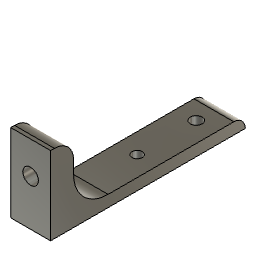
L Bracket v3 (Autodesk Fusion 360 design; units mm, degrees)
Autodesk Fusion 360 part; units mm, degrees
note: some values were not read from the file. Set by a fixed rule: which sketch regions a step uses.
sketch "Sketch1" plane through (0, 0, 0) normal (1, 0, 0) x (0, 1, 0)
  line L0 (0, 0) -> (0, 51)
  line L1 (0, 0) -> (127, 0)
  line L2 (127, 0) -> (127, 0.0001)
  line L3 (0, 51) -> (2.5, 51)
  line L4 (37.5, 7.5) -> (119.5, 7.5)
  line L5 (-5, 0) -> (-5, 33)
  line L6 (69.5, -10) -> (108, -10)
  line L7 (15, 30) -> (15, 38.5)
  arc A0 (15, 38.5) -> (2.5, 51) centre (2.5, 38.5) ccw
  arc A1 (127, 0.0001) -> (119.5, 7.5) centre (119.5, 0) ccw
  arc A2 (15, 30) -> (37.5, 7.5) centre (37.5, 30) ccw
  point P0 (126.9999, 7.5)
  point P1 (15, 51)
  point P2 (15, 7.5)
  dimension "d1" = 51
  dimension "d2" = 127
  dimension "d5" = 7.5
  dimension "d6" = 43.5
  dimension "d7" = 33
  dimension "d10" = 12.5
  dimension "d11" = 7.5
  dimension "d12" = 22.5
  constraint coincident L0.start L1.start
  constraint vertical L0
  constraint horizontal L1
  constraint perpendicular L0 L3
  constraint parallel L0 L5
  constraint perpendicular L3 L7
  constraint coincident P1 L3
  constraint coincident P1 L7
  constraint tangent L3 A0
  constraint tangent L7 A0
  constraint coincident P0 L2
  constraint coincident P0 L4
  constraint tangent L2 A1
  constraint tangent L4 A1
  constraint coincident P2 L4
  constraint coincident P2 L7
  constraint tangent L4 A2
  constraint tangent L7 A2
  measures "d1" distance of L0.start L0.end
  measures "d2" distance of L0.start L1.end
  measures "d5" distance of L1.end P0
  measures "d6" distance of P1 P2
  measures "d7" distance of L5.start L5.end
  measures "d10" radius of A0
  measures "d11" radius of A1
  measures "d12" radius of A2
sketch "Sketch2" plane through (0, 0, 0) normal (0, 0, 1) x (1, 0, 0)
  circle A0 centre (0, 69.5) radius 3.375
  circle A1 centre (0, 108) radius 3.875
  dimension "d13" = 6.75
  dimension "d14" = 7.75
  measures "d13" diameter of A0
  measures "d14" diameter of A1
sketch "Sketch3" plane through (0, 0, 0) normal (0, 1, 0) x (1, 0, 0)
  circle A0 centre (0, -30) radius 5.1
  circle A1 centre (0, -30) radius 11.15
  dimension "d15" = 10.2
  dimension "d16" = 22.3
  constraint concentric A0 A1
  measures "d15" diameter of A0
  measures "d16" diameter of A1
extrude "Extrude1" add sketch "Sketch1" along normal mid plane 26
extrude "Extrude2" cut sketch "Sketch2" along normal blind 20
extrude "Extrude3" cut sketch "Sketch3" along normal blind 90 contours A0
extrude "Extrude4" cut sketch "Sketch3" along normal blind 20 from surface at 8.2
named bodies: "FH L Bracket"
